oled_display (Autodesk Fusion 360 design; units mm, degrees)
Autodesk Fusion 360 part; units mm, degrees
sketch "Sketch1" plane through (0, 0, 0) normal (1, 0, 0) x (0, 1, 0)
  line L0 (0, 0) -> (-18.5, 0)
  line L1 (-18.5, 0) -> (-18.5, 31.5)
  line L2 (-18.5, 31.5) -> (0, 31.5)
  line L3 (0, 31.5) -> (0, 0)
  dimension "d1" = 18.5
  dimension "d2" = 31.5
  constraint horizontal L0
  constraint vertical L1
  constraint horizontal L2
  constraint vertical L3
  constraint coincident L0.start L3.end
  measures "d1" distance of L1.end L2.end
  measures "d2" distance of L0.end L1.end
extrude "Extrude1" add sketch "Sketch1" along normal blind 1.7
sketch "Sketch2" plane through (1.7, 0, 0) normal (1, 0, 0) x (0, 1, 0)
  line L0 (0, 31.5) -> (-18.5, 31.5)
  line L1 (-18.5, 31.5) -> (-18.5, 0)
  line L2 (-18.5, 0) -> (0, 0)
  line L3 (0, 0) -> (0, 31.5)
  line L4 (-12.8628, 25.99) -> (-5.7046, 25.99)
  line L5 (-5.7046, 25.99) -> (-5.7046, 21.1609)
  line L6 (-5.7046, 21.1609) -> (-6.5493, 21.1609)
  line L7 (-6.5493, 21.1609) -> (-6.5493, 25.0427)
  line L8 (-6.5493, 25.0427) -> (-8.7661, 25.0427)
  line L9 (-8.7661, 25.0427) -> (-8.7661, 21.6834)
  line L10 (-8.7661, 21.6834) -> (-9.6109, 21.6834)
  line L11 (-9.6109, 21.6834) -> (-9.6109, 25.0427)
  line L12 (-9.6109, 25.0427) -> (-12.8628, 25.0427)
  line L13 (-12.8628, 25.0427) -> (-12.8628, 25.99)
  line L14 (-12.8628, 20.0525) -> (-7.6773, 20.0525)
  line L15 (-7.6773, 20.0525) -> (-7.6773, 19.2615)
  line L16 (-7.6773, 19.2615) -> (-8.4634, 19.2615)
  spline S0 degree 3 poles (-8.4634, 19.2615) (-8.3037, 19.1734) (-8.032, 19.0235) (-7.8223, 18.7961) (-7.7359, 18.7024) knots 0 0 0 0 0.05425 0.092273 0.092273 0.092273 0.092273
  spline S1 degree 3 poles (-7.7359, 18.7024) (-7.6846, 18.615) (-7.5823, 18.4406) (-7.5675, 18.239) (-7.5601, 18.1384) knots 0 0 0 0 0.029972 0.059777 0.059777 0.059777 0.059777
  spline S2 degree 3 poles (-7.5601, 18.1384) (-7.5741, 17.9862) (-7.6037, 17.6653) (-7.7607, 17.3833) (-7.8433, 17.2351) knots 0 0 0 0 0.045356 0.095599 0.095599 0.095599 0.095599
  line L17 (-7.8433, 17.2351) -> (-8.6587, 17.5379)
  spline S3 degree 3 poles (-8.6587, 17.5379) (-8.6032, 17.643) (-8.4964, 17.8453) (-8.4774, 18.073) (-8.4683, 18.1824) knots 0 0 0 0 0.03525 0.067826 0.067826 0.067826 0.067826
  spline S4 degree 3 poles (-8.4683, 18.1824) (-8.4755, 18.276) (-8.4899, 18.463) (-8.5911, 18.621) (-8.6416, 18.7) knots 0 0 0 0 0.027685 0.055345 0.055345 0.055345 0.055345
  spline S5 degree 3 poles (-8.6416, 18.7) (-8.7065, 18.7714) (-8.8404, 18.9189) (-9.0266, 18.9903) (-9.1226, 19.0271) knots 0 0 0 0 0.028537 0.058895 0.058895 0.058895 0.058895
  spline S6 degree 3 poles (-9.1226, 19.0271) (-9.2853, 19.0698) (-9.6213, 19.1581) (-9.9687, 19.1683) (-10.148, 19.1736) knots 0 0 0 0 0.050287 0.103879 0.103879 0.103879 0.103879
  line L18 (-10.148, 19.1736) -> (-12.8628, 19.1736)
  line L19 (-12.8628, 19.1736) -> (-12.8628, 20.0525)
  spline S7 degree 3 poles (-10.27, 17.0398) (-9.8336, 17.0198) (-9.0308, 16.9829) (-8.4165, 16.4721) (-8.1363, 16.239) knots 0 0 0 0 0.126955 0.233506 0.233506 0.233506 0.233506
  spline S8 degree 3 poles (-8.1363, 16.239) (-7.9682, 16.0002) (-7.6241, 15.5111) (-7.5817, 14.9138) (-7.5601, 14.6082) knots 0 0 0 0 0.085882 0.175909 0.175909 0.175909 0.175909
  spline S9 degree 3 poles (-7.5601, 14.6082) (-7.5861, 14.2711) (-7.6369, 13.614) (-8.0564, 13.107) (-8.2608, 12.8601) knots 0 0 0 0 0.098734 0.192484 0.192484 0.192484 0.192484
  spline S10 degree 3 poles (-8.2608, 12.8601) (-8.5286, 12.6624) (-9.102, 12.2392) (-9.8162, 12.2015) (-10.1968, 12.1814) knots 0 0 0 0 0.097737 0.209205 0.209205 0.209205 0.209205
  spline S11 degree 3 poles (-10.1968, 12.1814) (-10.4988, 12.1873) (-11.042, 12.1978) (-11.5472, 12.3944) (-11.7715, 12.4817) knots 0 0 0 0 0.089731 0.161415 0.161415 0.161415 0.161415
  spline S12 degree 3 poles (-11.7715, 12.4817) (-11.9522, 12.5935) (-12.3149, 12.8179) (-12.5465, 13.176) (-12.6626, 13.3557) knots 0 0 0 0 0.0629 0.126218 0.126218 0.126218 0.126218
  spline S13 degree 3 poles (-12.6626, 13.3557) (-12.7552, 13.5523) (-12.942, 13.9492) (-12.9673, 14.3872) (-12.98, 14.6082) knots 0 0 0 0 0.064547 0.130274 0.130274 0.130274 0.130274
  spline S14 degree 3 poles (-12.98, 14.6082) (-12.9549, 14.9497) (-12.9064, 15.6111) (-12.4854, 16.1216) (-12.2818, 16.3684) knots 0 0 0 0 0.099985 0.193582 0.193582 0.193582 0.193582
  spline S15 degree 3 poles (-12.2818, 16.3684) (-12.0075, 16.5639) (-11.4084, 16.9907) (-10.6702, 17.0226) (-10.27, 17.0398) knots 0 0 0 0 0.098972 0.216147 0.216147 0.216147 0.216147
  spline S16 degree 3 poles (-10.27, 16.1365) (-10.5691, 16.128) (-11.1069, 16.1128) (-11.5604, 15.8283) (-11.7617, 15.7019) knots 0 0 0 0 0.087772 0.157881 0.157881 0.157881 0.157881
  spline S17 degree 3 poles (-11.7617, 15.7019) (-11.9063, 15.5477) (-12.1954, 15.2393) (-12.2367, 14.8185) (-12.2573, 14.6082) knots 0 0 0 0 0.061561 0.123123 0.123123 0.123123 0.123123
  spline S18 degree 3 poles (-12.2573, 14.6082) (-12.2364, 14.399) (-12.1942, 13.9795) (-11.9046, 13.673) (-11.7593, 13.5193) knots 0 0 0 0 0.061216 0.122791 0.122791 0.122791 0.122791
  spline S19 degree 3 poles (-11.7593, 13.5193) (-11.5552, 13.393) (-11.0927, 13.1068) (-10.5461, 13.0926) (-10.2407, 13.0847) knots 0 0 0 0 0.070813 0.160463 0.160463 0.160463 0.160463
  spline S20 degree 3 poles (-10.2407, 13.0847) (-9.9503, 13.0942) (-9.4234, 13.1115) (-8.9816, 13.3946) (-8.7832, 13.5217) knots 0 0 0 0 0.085237 0.154677 0.154677 0.154677 0.154677
  spline S21 degree 3 poles (-8.7832, 13.5217) (-8.6387, 13.6757) (-8.351, 13.9822) (-8.3087, 14.4002) (-8.2876, 14.6082) knots 0 0 0 0 0.061512 0.122417 0.122417 0.122417 0.122417
  spline S22 degree 3 poles (-8.2876, 14.6082) (-8.3081, 14.8185) (-8.349, 15.2388) (-8.6369, 15.5476) (-8.7808, 15.7019) knots 0 0 0 0 0.06155 0.123001 0.123001 0.123001 0.123001
  spline S23 degree 3 poles (-8.7808, 15.7019) (-8.9815, 15.8283) (-9.434, 16.113) (-9.9712, 16.1281) (-10.27, 16.1365) knots 0 0 0 0 0.069947 0.157659 0.157659 0.157659 0.157659
  line L20 (-12.8628, 11.1511) -> (-7.6773, 11.1511)
  line L21 (-7.6773, 11.1511) -> (-7.6773, 10.3601)
  line L22 (-7.6773, 10.3601) -> (-8.4146, 10.3601)
  spline S24 degree 3 poles (-8.4146, 10.3601) (-8.1654, 10.146) (-7.6596, 9.7113) (-7.5936, 9.0468) (-7.5601, 8.7097) knots 0 0 0 0 0.094776 0.192358 0.192358 0.192358 0.192358
  spline S25 degree 3 poles (-7.5601, 8.7097) (-7.5664, 8.5583) (-7.5788, 8.2623) (-7.6794, 7.9839) (-7.7285, 7.8479) knots 0 0 0 0 0.04518 0.088272 0.088272 0.088272 0.088272
  spline S26 degree 3 poles (-7.7285, 7.8479) (-7.7858, 7.7275) (-7.8936, 7.5012) (-8.0821, 7.3366) (-8.1704, 7.2595) knots 0 0 0 0 0.039495 0.074282 0.074282 0.074282 0.074282
  spline S27 degree 3 poles (-8.1704, 7.2595) (-8.2679, 7.1989) (-8.4697, 7.0733) (-8.7005, 7.0158) (-8.8198, 6.9861) knots 0 0 0 0 0.034206 0.07085 0.07085 0.07085 0.07085
  spline S28 degree 3 poles (-8.8198, 6.9861) (-8.9316, 6.972) (-9.2152, 6.9363) (-9.5011, 6.9369) (-9.6743, 6.9373) knots 0 0 0 0 0.033768 0.085663 0.085663 0.085663 0.085663
  line L23 (-9.6743, 6.9373) -> (-12.8628, 6.9373)
  line L24 (-12.8628, 6.9373) -> (-12.8628, 7.8162)
  line L25 (-12.8628, 7.8162) -> (-9.7085, 7.8162)
  spline S29 degree 3 poles (-9.7085, 7.8162) (-9.551, 7.817) (-9.2786, 7.8185) (-9.016, 7.889) (-8.9053, 7.9187) knots 0 0 0 0 0.047006 0.081267 0.081267 0.081267 0.081267
  spline S30 degree 3 poles (-8.9053, 7.9187) (-8.8206, 7.9603) (-8.6479, 8.0451) (-8.537, 8.2024) (-8.4805, 8.2825) knots 0 0 0 0 0.027833 0.056732 0.056732 0.056732 0.056732
  spline S31 degree 3 poles (-8.4805, 8.2825) (-8.4342, 8.3753) (-8.3381, 8.5682) (-8.3274, 8.7836) (-8.3218, 8.8953) knots 0 0 0 0 0.030776 0.063912 0.063912 0.063912 0.063912
  spline S32 degree 3 poles (-8.3218, 8.8953) (-8.336, 9.0753) (-8.3643, 9.4319) (-8.5743, 9.7213) (-8.6782, 9.8645) knots 0 0 0 0 0.053061 0.105073 0.105073 0.105073 0.105073
  spline S33 degree 3 poles (-8.6782, 9.8645) (-8.8449, 9.9826) (-9.2454, 10.2665) (-9.7412, 10.2701) (-10.0308, 10.2722) knots 0 0 0 0 0.060011 0.144248 0.144248 0.144248 0.144248
  line L26 (-10.0308, 10.2722) -> (-12.8628, 10.2722)
  line L27 (-12.8628, 10.2722) -> (-12.8628, 11.1511)
  line L28 (-12.0767, 3.6707) -> (-12.853, 3.5437)
  spline S34 degree 3 poles (-12.853, 3.5437) (-12.8758, 3.6605) (-12.9186, 3.88) (-12.9272, 4.1033) (-12.9312, 4.2078) knots 0 0 0 0 0.035641 0.066952 0.066952 0.066952 0.066952
  spline S35 degree 3 poles (-12.9312, 4.2078) (-12.9284, 4.3515) (-12.9235, 4.6089) (-12.8238, 4.8455) (-12.7798, 4.95) knots 0 0 0 0 0.042649 0.076356 0.076356 0.076356 0.076356
  spline S36 degree 3 poles (-12.7798, 4.95) (-12.7268, 5.0307) (-12.6242, 5.187) (-12.4609, 5.2774) (-12.3819, 5.3211) knots 0 0 0 0 0.028484 0.055146 0.055146 0.055146 0.055146
  spline S37 degree 3 poles (-12.3819, 5.3211) (-12.2548, 5.3519) (-11.9148, 5.4346) (-11.564, 5.4308) (-11.3443, 5.4285) knots 0 0 0 0 0.039108 0.104654 0.104654 0.104654 0.104654
  line L29 (-11.3443, 5.4285) -> (-8.3609, 5.4285)
  line L30 (-8.3609, 5.4285) -> (-8.3609, 6.073)
  line L31 (-8.3609, 6.073) -> (-7.6773, 6.073)
  line L32 (-7.6773, 6.073) -> (-7.6773, 5.4285)
  line L33 (-7.6773, 5.4285) -> (-6.3931, 5.4285)
  line L34 (-6.3931, 5.4285) -> (-5.8657, 4.5545)
  line L35 (-5.8657, 4.5545) -> (-7.6773, 4.5545)
  line L36 (-7.6773, 4.5545) -> (-7.6773, 3.6707)
  line L37 (-7.6773, 3.6707) -> (-8.3609, 3.6707)
  line L38 (-8.3609, 3.6707) -> (-8.3609, 4.5545)
  line L39 (-8.3609, 4.5545) -> (-11.3931, 4.5545)
  spline S38 degree 3 poles (-11.3931, 4.5545) (-11.4966, 4.5558) (-11.6598, 4.5578) (-11.8185, 4.5214) (-11.8765, 4.5081) knots 0 0 0 0 0.030906 0.048705 0.048705 0.048705 0.048705
  spline S39 degree 3 poles (-11.8765, 4.5081) (-11.9106, 4.4899) (-11.9797, 4.4532) (-12.0246, 4.3892) (-12.0474, 4.3567) knots 0 0 0 0 0.011413 0.023119 0.023119 0.023119 0.023119
  spline S40 degree 3 poles (-12.0474, 4.3567) (-12.0658, 4.3148) (-12.1078, 4.2194) (-12.1098, 4.1149) (-12.1109, 4.0564) knots 0 0 0 0 0.013616 0.030961 0.030961 0.030961 0.030961
  spline S41 degree 3 poles (-12.1109, 4.0564) (-12.1088, 3.9998) (-12.1043, 3.8706) (-12.0866, 3.7426) (-12.0767, 3.6707) knots 0 0 0 0 0.016989 0.038747 0.038747 0.038747 0.038747
extrude "Extrude2" add sketch "Sketch2" along normal blind 1 contours L4 L5 L6 L7 L8 L9 L10 L11 L12 L13 | L14 L15 L16 S0 S1 S2 L17 S3 S4 S5 S6 L18 L19 | S7 S8 S9 S10 S11 S12 S13 S14 S15 | L20 L21 L22 S24 S25 S26 S27 S28 L23 L24 L25 S29 S30 S31 S32 S33 L26 L27 | L28 S34 S35 S36 S37 L29 L30 L31 L32 L33 L34 L35 L36 L37 L38 L39 S38 S39 S40 S41
sketch "Sketch3" plane through (0, 0, 31.5) normal (0, 0, 1) x (-1, 0, 0)
  line L0 (0, 0) -> (0, 18.5)
  line L1 (0, 18.5) -> (-1.7, 18.5)
  line L2 (-1.7, 18.5) -> (-1.7, 0)
  line L3 (-1.7, 0) -> (0, 0)
  line L4 (-0.5, 2.5) -> (-1.7, 2.5)
  line L5 (-1.7, 2.5) -> (-1.7, 13.5)
  line L6 (-1.7, 13.5) -> (-0.5, 13.5)
  line L7 (-0.5, 13.5) -> (-0.5, 2.5)
  dimension "d7" = 5
  dimension "d8" = 2.5
  dimension "d9" = 0.5
  constraint horizontal L4
  constraint vertical L5
  constraint horizontal L6
  constraint vertical L7
  constraint coincident L2 L5.end
  measures "d7" distance of L1 L6
  measures "d8" distance of L3 L4
  measures "d9" distance of L0 L7
extrude "Extrude3" add sketch "Sketch3" along normal blind 1.6 contours L2 L4 L5 L6 L7
sketch "Sketch4" plane through (1.7, 0, 0) normal (1, 0, 0) x (0, 1, 0)
  spline S0 degree 3 poles (-12.1109, 4.0564) (-12.1088, 3.9998) (-12.1043, 3.8706) (-12.0866, 3.7426) (-12.0767, 3.6707) knots 0 0 0 0 0.016989 0.038747 0.038747 0.038747 0.038747
  line L0 (-12.0767, 3.6707) -> (-12.853, 3.5437)
  spline S1 degree 3 poles (-12.853, 3.5437) (-12.8758, 3.6605) (-12.9186, 3.88) (-12.9272, 4.1033) (-12.9312, 4.2078) knots 0 0 0 0 0.035641 0.066952 0.066952 0.066952 0.066952
  spline S2 degree 3 poles (-12.9312, 4.2078) (-12.9284, 4.3515) (-12.9235, 4.6089) (-12.8238, 4.8455) (-12.7798, 4.95) knots 0 0 0 0 0.042649 0.076356 0.076356 0.076356 0.076356
  spline S3 degree 3 poles (-12.7798, 4.95) (-12.7268, 5.0307) (-12.6242, 5.187) (-12.4609, 5.2774) (-12.3819, 5.3211) knots 0 0 0 0 0.028484 0.055146 0.055146 0.055146 0.055146
  spline S4 degree 3 poles (-12.3819, 5.3211) (-12.2548, 5.3519) (-11.9148, 5.4346) (-11.564, 5.4308) (-11.3443, 5.4285) knots 0 0 0 0 0.039108 0.104654 0.104654 0.104654 0.104654
  line L1 (-11.3443, 5.4285) -> (-8.3609, 5.4285)
  line L2 (-8.3609, 5.4285) -> (-8.3609, 6.073)
  line L3 (-8.3609, 6.073) -> (-7.6773, 6.073)
  line L4 (-7.6773, 6.073) -> (-7.6773, 5.4285)
  line L5 (-7.6773, 5.4285) -> (-6.3931, 5.4285)
  line L6 (-6.3931, 5.4285) -> (-5.8657, 4.5545)
  line L7 (-5.8657, 4.5545) -> (-7.6773, 4.5545)
  line L8 (-7.6773, 4.5545) -> (-7.6773, 3.6707)
  line L9 (-7.6773, 3.6707) -> (-8.3609, 3.6707)
  line L10 (-8.3609, 3.6707) -> (-8.3609, 4.5545)
  line L11 (-8.3609, 4.5545) -> (-11.3931, 4.5545)
  spline S5 degree 3 poles (-11.3931, 4.5545) (-11.4966, 4.5558) (-11.6598, 4.5578) (-11.8185, 4.5214) (-11.8765, 4.5081) knots 0 0 0 0 0.030906 0.048705 0.048705 0.048705 0.048705
  spline S6 degree 3 poles (-11.8765, 4.5081) (-11.9106, 4.4899) (-11.9797, 4.4532) (-12.0246, 4.3892) (-12.0474, 4.3567) knots 0 0 0 0 0.011413 0.023119 0.023119 0.023119 0.023119
  spline S7 degree 3 poles (-12.0474, 4.3567) (-12.0658, 4.3148) (-12.1078, 4.2194) (-12.1098, 4.1149) (-12.1109, 4.0564) knots 0 0 0 0 0.013616 0.030961 0.030961 0.030961 0.030961
  line L12 (-12.8628, 25.0427) -> (-12.8628, 25.99)
  line L13 (-12.8628, 25.99) -> (-5.7046, 25.99)
  line L14 (-5.7046, 25.99) -> (-5.7046, 21.1609)
  line L15 (-5.7046, 21.1609) -> (-6.5493, 21.1609)
  line L16 (-6.5493, 21.1609) -> (-6.5493, 25.0427)
  line L17 (-6.5493, 25.0427) -> (-8.7661, 25.0427)
  line L18 (-8.7661, 25.0427) -> (-8.7661, 21.6834)
  line L19 (-8.7661, 21.6834) -> (-9.6109, 21.6834)
  line L20 (-9.6109, 21.6834) -> (-9.6109, 25.0427)
  line L21 (-9.6109, 25.0427) -> (-12.8628, 25.0427)
  line L22 (-12.8628, 10.2722) -> (-12.8628, 11.1511)
  line L23 (-12.8628, 11.1511) -> (-7.6773, 11.1511)
  line L24 (-7.6773, 11.1511) -> (-7.6773, 10.3601)
  line L25 (-7.6773, 10.3601) -> (-8.4146, 10.3601)
  spline S8 degree 3 poles (-8.4146, 10.3601) (-8.1654, 10.146) (-7.6596, 9.7113) (-7.5936, 9.0468) (-7.5601, 8.7097) knots 0 0 0 0 0.094776 0.192358 0.192358 0.192358 0.192358
  spline S9 degree 3 poles (-7.5601, 8.7097) (-7.5664, 8.5583) (-7.5788, 8.2623) (-7.6794, 7.9839) (-7.7285, 7.8479) knots 0 0 0 0 0.04518 0.088272 0.088272 0.088272 0.088272
  spline S10 degree 3 poles (-7.7285, 7.8479) (-7.7858, 7.7275) (-7.8936, 7.5012) (-8.0821, 7.3366) (-8.1704, 7.2595) knots 0 0 0 0 0.039495 0.074282 0.074282 0.074282 0.074282
  spline S11 degree 3 poles (-8.1704, 7.2595) (-8.2679, 7.1989) (-8.4697, 7.0733) (-8.7005, 7.0158) (-8.8198, 6.9861) knots 0 0 0 0 0.034206 0.07085 0.07085 0.07085 0.07085
  spline S12 degree 3 poles (-8.8198, 6.9861) (-8.9316, 6.972) (-9.2152, 6.9363) (-9.5011, 6.9369) (-9.6743, 6.9373) knots 0 0 0 0 0.033768 0.085663 0.085663 0.085663 0.085663
  line L26 (-9.6743, 6.9373) -> (-12.8628, 6.9373)
  line L27 (-12.8628, 6.9373) -> (-12.8628, 7.8162)
  line L28 (-12.8628, 7.8162) -> (-9.7085, 7.8162)
  spline S13 degree 3 poles (-9.7085, 7.8162) (-9.551, 7.817) (-9.2786, 7.8185) (-9.016, 7.889) (-8.9053, 7.9187) knots 0 0 0 0 0.047006 0.081267 0.081267 0.081267 0.081267
  spline S14 degree 3 poles (-8.9053, 7.9187) (-8.8206, 7.9603) (-8.6479, 8.0451) (-8.537, 8.2024) (-8.4805, 8.2825) knots 0 0 0 0 0.027833 0.056732 0.056732 0.056732 0.056732
  spline S15 degree 3 poles (-8.4805, 8.2825) (-8.4342, 8.3753) (-8.3381, 8.5682) (-8.3274, 8.7836) (-8.3218, 8.8953) knots 0 0 0 0 0.030776 0.063912 0.063912 0.063912 0.063912
  spline S16 degree 3 poles (-8.3218, 8.8953) (-8.336, 9.0753) (-8.3643, 9.4319) (-8.5743, 9.7213) (-8.6782, 9.8645) knots 0 0 0 0 0.053061 0.105073 0.105073 0.105073 0.105073
  spline S17 degree 3 poles (-8.6782, 9.8645) (-8.8449, 9.9826) (-9.2454, 10.2665) (-9.7412, 10.2701) (-10.0308, 10.2722) knots 0 0 0 0 0.060011 0.144248 0.144248 0.144248 0.144248
  line L29 (-10.0308, 10.2722) -> (-12.8628, 10.2722)
  line L30 (-12.8628, 19.1736) -> (-12.8628, 20.0525)
  line L31 (-12.8628, 20.0525) -> (-7.6773, 20.0525)
  line L32 (-7.6773, 20.0525) -> (-7.6773, 19.2615)
  line L33 (-7.6773, 19.2615) -> (-8.4634, 19.2615)
  spline S18 degree 3 poles (-8.4634, 19.2615) (-8.3037, 19.1734) (-8.032, 19.0235) (-7.8223, 18.7961) (-7.7359, 18.7024) knots 0 0 0 0 0.05425 0.092273 0.092273 0.092273 0.092273
  spline S19 degree 3 poles (-7.7359, 18.7024) (-7.6846, 18.615) (-7.5823, 18.4406) (-7.5675, 18.239) (-7.5601, 18.1384) knots 0 0 0 0 0.029972 0.059777 0.059777 0.059777 0.059777
  spline S20 degree 3 poles (-7.5601, 18.1384) (-7.5741, 17.9862) (-7.6037, 17.6653) (-7.7607, 17.3833) (-7.8433, 17.2351) knots 0 0 0 0 0.045356 0.095599 0.095599 0.095599 0.095599
  line L34 (-7.8433, 17.2351) -> (-8.6587, 17.5379)
  spline S21 degree 3 poles (-8.6587, 17.5379) (-8.6032, 17.643) (-8.4964, 17.8453) (-8.4774, 18.073) (-8.4683, 18.1824) knots 0 0 0 0 0.03525 0.067826 0.067826 0.067826 0.067826
  spline S22 degree 3 poles (-8.4683, 18.1824) (-8.4755, 18.276) (-8.4899, 18.463) (-8.5911, 18.621) (-8.6416, 18.7) knots 0 0 0 0 0.027685 0.055345 0.055345 0.055345 0.055345
  spline S23 degree 3 poles (-8.6416, 18.7) (-8.7065, 18.7714) (-8.8404, 18.9189) (-9.0266, 18.9903) (-9.1226, 19.0271) knots 0 0 0 0 0.028537 0.058895 0.058895 0.058895 0.058895
  spline S24 degree 3 poles (-9.1226, 19.0271) (-9.2853, 19.0698) (-9.6213, 19.1581) (-9.9687, 19.1683) (-10.148, 19.1736) knots 0 0 0 0 0.050287 0.103879 0.103879 0.103879 0.103879
  line L35 (-10.148, 19.1736) -> (-12.8628, 19.1736)
  line L36 (0, 31.5) -> (-2.5, 31.5)
  line L37 (-2.5, 31.5) -> (-2.5, 33.1)
  line L38 (-2.5, 33.1) -> (-13.5, 33.1)
  line L39 (-13.5, 33.1) -> (-13.5, 31.5)
  line L40 (-13.5, 31.5) -> (-18.5, 31.5)
  line L41 (-18.5, 31.5) -> (-18.5, 0)
  line L42 (-18.5, 0) -> (0, 0)
  line L43 (0, 0) -> (0, 31.5)
  spline S25 degree 3 poles (-12.2818, 16.3684) (-12.0075, 16.5639) (-11.4084, 16.9907) (-10.6702, 17.0226) (-10.27, 17.0398) knots 0 0 0 0 0.098972 0.216147 0.216147 0.216147 0.216147
  spline S26 degree 3 poles (-10.27, 17.0398) (-9.8336, 17.0198) (-9.0308, 16.9829) (-8.4165, 16.4721) (-8.1363, 16.239) knots 0 0 0 0 0.126955 0.233506 0.233506 0.233506 0.233506
  spline S27 degree 3 poles (-8.1363, 16.239) (-7.9682, 16.0002) (-7.6241, 15.5111) (-7.5817, 14.9138) (-7.5601, 14.6082) knots 0 0 0 0 0.085882 0.175909 0.175909 0.175909 0.175909
  spline S28 degree 3 poles (-7.5601, 14.6082) (-7.5861, 14.2711) (-7.6369, 13.614) (-8.0564, 13.107) (-8.2608, 12.8601) knots 0 0 0 0 0.098734 0.192484 0.192484 0.192484 0.192484
  spline S29 degree 3 poles (-8.2608, 12.8601) (-8.5286, 12.6624) (-9.102, 12.2392) (-9.8162, 12.2015) (-10.1968, 12.1814) knots 0 0 0 0 0.097737 0.209205 0.209205 0.209205 0.209205
  spline S30 degree 3 poles (-10.1968, 12.1814) (-10.4988, 12.1873) (-11.042, 12.1978) (-11.5472, 12.3944) (-11.7715, 12.4817) knots 0 0 0 0 0.089731 0.161415 0.161415 0.161415 0.161415
  spline S31 degree 3 poles (-11.7715, 12.4817) (-11.9522, 12.5935) (-12.3149, 12.8179) (-12.5465, 13.176) (-12.6626, 13.3557) knots 0 0 0 0 0.0629 0.126218 0.126218 0.126218 0.126218
  spline S32 degree 3 poles (-12.6626, 13.3557) (-12.7552, 13.5523) (-12.942, 13.9492) (-12.9673, 14.3872) (-12.98, 14.6082) knots 0 0 0 0 0.064547 0.130274 0.130274 0.130274 0.130274
  spline S33 degree 3 poles (-12.98, 14.6082) (-12.9549, 14.9497) (-12.9064, 15.6111) (-12.4854, 16.1216) (-12.2818, 16.3684) knots 0 0 0 0 0.099985 0.193582 0.193582 0.193582 0.193582
  line L44 (-18.5, 31.5) -> (0, 31.5)
  line L45 (0, 31.5) -> (0, 28.6)
  line L46 (0, 28.6) -> (-18.5, 28.6)
  line L47 (-18.5, 28.6) -> (-18.5, 31.5)
  line L48 (-18.5, 31.5) -> (0, 31.5)
  line L49 (0, 31.5) -> (0, 34.5)
  line L50 (0, 34.5) -> (-18.5, 34.5)
  line L51 (-18.5, 34.5) -> (-18.5, 31.5)
  dimension "d12" = 2.9
  constraint horizontal L44
  constraint vertical L45
  constraint horizontal L46
  constraint vertical L47
  constraint coincident L43 L45.end
  constraint coincident L40.end L41.start
  constraint horizontal L48
  constraint vertical L49
  constraint horizontal L50
  constraint vertical L51
  measures "d12" distance of L36.start L45.end
extrude "Extrude4" add sketch "Sketch4" along normal blind 0.1 contours L36 L40 L41 L43 L44 L45 L46 L47 L48 | L37 L38 L39 L44 L48
